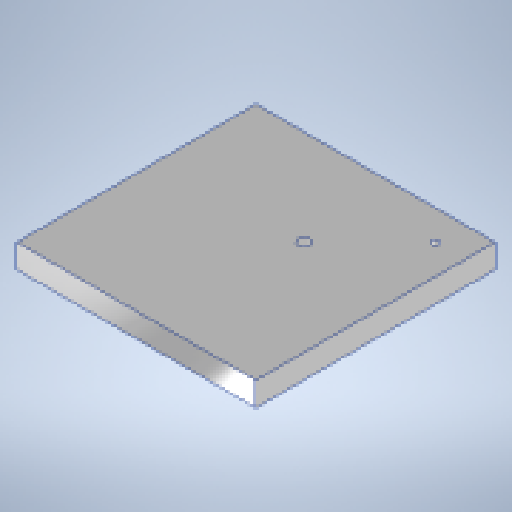
# Autodesk Inventor part: base_plate6
Saved by Autodesk Inventor 2024 (Build 280153000, 153)
## iProperties
Created: 2025-02-22
Part Number: base_plate6
Material: アルミニウム 6061
Document SubType Name: Modeling
Designer: tanoue_kota
Density: 2.7 g/cm^3
Appearance: アルミニウム - フラット
Author: tanoue_kota
Autodesk Inventor part; units mm, degrees
ref_plane "YZ Plane" through (0, 0, 0) normal (1, 0, 0) x (0, 1, 0)
ref_plane "XZ Plane" through (0, 0, 0) normal (0, 1, 0) x (-1, 0, 0)
ref_plane "XY Plane" through (0, 0, 0) normal (0, 0, 1) x (1, 0, 0)
sketch "スケッチ1" plane through (0, 0, 0) normal (0, 1, 0) x (-1, 0, 0)
  line L0 (0, 0) -> (100, 0)
  line L1 (100, 0) -> (100, 100)
  line L2 (100, 100) -> (0, 100)
  line L3 (0, 100) -> (0, 0)
  dimension "d0" = 100
  dimension "d1" = 100
  constraints: 8 end point, 2 parallel, 1 horizontal, 1 perpendicular
  measures "d0" distance of L0.start L0.end
  measures "d1" distance of L2.end L0.start
extrude "押し出し1" add sketch "スケッチ1" along normal blind 10
sketch "スケッチ2" plane through (0, 10, 0) normal (0, 1, 0) x (1, 0, 0)
  line L0 (0, 0) -> (-100, 0) projected
  line L1 (0, 0) -> (-40, 0)
  line L2 (-40, 0) -> (-40, -40)
  line L3 (-40, -40) -> (0, -40)
  line L4 (0, -40) -> (0, 0)
  dimension "d4" = 40
  dimension "d5" = 40
  constraints: 8 end point, 2 parallel, 1 coincident, 1 horizontal, 1 perpendicular
  measures "d4" distance of L1.end L2.end
  measures "d5" distance of L2.end L3.end
hole "穴1" at (-40, 10, 40) direction (0, -1, 0) diameter 4.917 end through all thread size "M6x1" class "6H" standard "ISO Metric profile"
sketch "スケッチ3" plane through (0, 10, 0) normal (0, 1, 0) x (1, 0, 0)
  circle A0 centre (-40, -40) radius 2.4585 projected
  circle A1 centre (-40, -40) radius 39
  line L0 (-40, -40) -> (0, 0)
  point P0 (-12.4228, -12.4228)
  dimension "d23" = 78
  constraints: 2 end point, 1 coincident, 1 point on line, 3 other
hole "穴2" at (-12.4228, 10, 12.4228) direction (0, -1, 0) diameter 3.2 end through all
sketch "スケッチ4" plane through (0, 0, 0) normal (0, -1, 0) x (1, 0, 0)
  circle A0 centre (-12.4228, 12.4228) radius 1.6 projected
  circle A1 centre (-12.4228, 12.4228) radius 3
  point P0 (0, 0)
  dimension "d24" = 6
  constraints: 1 centre point, 1 coincident
  measures "d24" diameter of A1
extrude "押し出し2" cut sketch "スケッチ4" against normal blind 3.2 contours A0 | A1
